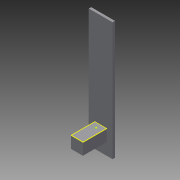
# Autodesk Inventor part: base
Saved by Autodesk Inventor 2014 SP1 (Build 180222100, 222)
## iProperties
Created: 2014-01-31
Part Number: base
Material: Generic
Document SubType Name: Modeling
Designer: Michael
Density: 1 g/cm^3
Appearance: Default
Author: Michael
Autodesk Inventor part; units mm, degrees
ref_plane "YZ Plane" through (0, 0, 0) normal (1, 0, 0) x (0, 1, 0)
ref_plane "XZ Plane" through (0, 0, 0) normal (0, 1, 0) x (-1, 0, 0)
ref_plane "XY Plane" through (0, 0, 0) normal (0, 0, 1) x (1, 0, 0)
sketch "Sketch1" plane through (0, 0, 0) normal (0, 0, 1) x (1, 0, 0)
  line L0 (-127, 635) -> (127, 635)
  line L1 (127, 635) -> (127, -635)
  line L2 (127, -635) -> (-127, -635)
  line L3 (-127, -635) -> (-127, 635)
  line L4 (-127, 635) -> (127, -635) construction
  line L5 (127, 635) -> (-127, -635) construction
  point P0 (0, 0)
  dimension "d0" = 254
  dimension "d1" = 1270
  constraints: 12 end point, 2 midpoint, 2 parallel, 1 horizontal, 1 perpendicular
  measures "d0" distance of L1.end L2.end
  measures "d1" distance of L0.end L1.end
extrude "Extrusion1" add sketch "Sketch1" along normal blind 25.4
sketch "Sketch2" plane through (0, 0, 25.4) normal (0, 0, 1) x (1, 0, 0)
  line L0 (127, 635) -> (-127, 635) projected
  line L1 (-63.5, -381) -> (63.5, -381)
  line L2 (63.5, -381) -> (63.5, -508)
  line L3 (63.5, -508) -> (-63.5, -508)
  line L4 (-63.5, -508) -> (-63.5, -381)
  line L5 (-63.5, -381) -> (63.5, -508) construction
  line L6 (63.5, -381) -> (-63.5, -508) construction
  line L7 (0, 635) -> (0, 508)
  point P0 (0, 0)
  dimension "d5" = 127
  dimension "d6" = 127
  dimension "d7" = 127
  constraints: 14 end point, 3 parallel, 1 horizontal, 1 midpoint, 1 perpendicular
  measures "d5" distance of L2.end L3.end
  measures "d6" distance of L1.end L2.end
  measures "d7" distance of L7.start L7.end
hole "Hole1" at (0, 508, 25.4) direction (0, 0, -1) diameter 6.35 end through all
extrude "Extrusion2" add sketch "Sketch2" along normal blind 254
sketch "Sketch3" plane through (-63.5, -381, 25.4) normal (0, 1, 0) x (1, 0, 0)
  line L0 (127, -254) -> (0, -254) projected
  line L1 (127, 0) -> (127, -254) projected
  line L2 (63.5, -254) -> (63.5, -50.8)
  point P0 (63.5, 25.4)
  dimension "d17" = 203.2
  constraints: 2 end point, 1 midpoint, 1 parallel
  measures "d17" distance of L2.start L2.end
hole "Hole2" at (0, -381, 76.2) direction (0, -1, 0) diameter 6.35 end through all
sketch "Sketch4" plane through (-63.5, -381, 25.4) normal (0, 1, 0) x (1, 0, 0)
  circle A0 centre (63.5, -50.8) radius 3.175 projected
  line L0 (0, 0) -> (127, 0) projected
  line L1 (0, 0) -> (0, -254) projected
  line L2 (127, -254) -> (0, -254) projected
  line L3 (127, 0) -> (127, -254) projected
  point P0 (63.5, 25.4)
  point P1 (63.5, -53.975)
  constraints: 1 vertical alignment, 1 other
body "Solid1"
